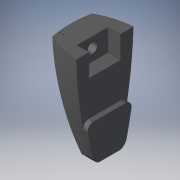
# Autodesk Inventor part: SCHUNK-1012602-FIN Co-act EGP 40/12
Saved by Autodesk Inventor 2019 (Build 230136000, 136)
## iProperties
Created: 2022-08-31
Part Number: SCHUNK-1012602-FIN Co-act EGP 40/12
Material: Generic
Catalog Web Link: www.cadenas.de
Description: FIN Co-act EGP-Finger Co-act EGP
Vendor: SCHUNK
Document SubType Name: Modeling
Designer: psAdmin
Manufacturer: SCHUNK
Mass: 14.2993 g
Surface Area: 56.9763 cm^2
Volume: 14.2993 cm^3
Density: 1 g/cm^3
Appearance: PSOLRGB-229-229-229
Category: PARTsolutions
Company: SCHUNK
Title: SCHUNK-1012602-FIN Co-act EGP 40/12
Author: Cadenas PARTsolutions
Comments: Finger Co-act EGP
PSOL_IDENT_0: {$CADENAS_DATA/23d-libs/schunk/greifsysteme/greifmodule/co_act/co_act_egp_c/fin_co_act_egp.prj},218
PSOL_IDENT_1: {VTYP=3D},{NB=SCHUNK-1012602-FIN Co-act EGP 40/12},{LINA=SCHUNK-1012602-FIN Co-act EGP 40/12},{NN=FI
PSOL_IDENT_2: N Co-act EGP},{DATE=21.12.2021 12:22:33},{GEOMDATE=21.11.2019 10:27:04},{VERSION=},{LINEID=30},{WBVA
PSOL_IDENT_3: R=},{WBNUMERIC=}  {NB=SCHUNK-1012602-FIN Co-act EGP 40/12},{LINA=SCHUNK-1012602-FIN Co-act EGP 40/12
PSOL_IDENT_4: },{KT=DUMMY},{IDNR=1012602},{TYP=FIN Co-act EGP 40/12},{TYP1=1.000},{R1=96.286},{L1=14.000},{A1=20.5
PSOL_IDENT_5: 00},{A2=0.000},{A3=0.000},{PARTSERVER=1},{B=0.000},{ANFGPKTEGH=0.000}
NB: SCHUNK-1012602-FIN Co-act EGP 40/12
NN: FIN Co-act EGP
NT: Finger Co-act EGP
NBSYN: SCHUNK-$IDNR.-$TYP.
LINA: SCHUNK-1012602-FIN Co-act EGP 40/12
CATALOG: SCHUNK
IDNR: 1012602
TYP: FIN Co-act EGP 40/12
TYP1: 1
R1: 96.286
L1: 14
A1: 20.5
A2: 0
A3: 0
PARTSERVER: 1
B: 0
ANFGPKTEGH: 0
SUPPLIER: SCHUNK
ARTICLENO: SCHUNK-1012602-FIN Co-act EGP 40/12
BOMINFO: SCHUNK-1012602-FIN Co-act EGP 40/12
CREATOR: CADENAS GmbH
Autodesk Inventor part; units mm, degrees
sketch "Sketch_1" plane through (0, 0, 0) normal (0, 0, 1) x (1, 0, 0)
  line L0 (0, 50) -> (0, 0)
  line L1 (0, 0) -> (20.15, 0)
  arc A0 (20.15, 0) -> (20.5, 0.35) centre (20.15, 0.35) ccw
  line L2 (20.5, 0.35) -> (20.5, 50)
  line L3 (20.5, 50) -> (0, 50)
  constraints: 8 end point, 2 point on circle, 1 centre point
extrude "Extrusion1" add sketch "Sketch_1" along normal mid plane 30
sketch "Sketch_2" plane through (0, 0, 0) normal (0, 0, 1) x (1, 0, 0)
  line L0 (18, 50) -> (18, 20.0436)
  line L1 (18, 20.0436) -> (20.5, 20)
  line L2 (20.5, 20) -> (20.5, 50)
  line L3 (20.5, 50) -> (18, 50)
  constraints: 8 end point
extrude "Extrusion2" cut sketch "Sketch_2" along normal mid plane 30
sketch "Sketch_4" plane through (0, 0, 0) normal (0, 0, 1) x (1, 0, 0)
  line L0 (49.5, 60) -> (49.5, -60)
  line L1 (-6, 50) -> (-6, 0)
  line L2 (-6, 0) -> (14, 0)
  arc A0 (0, 50) -> (14, 0) centre (96.286, 50.0001) ccw
  line L3 (0, 50) -> (-6, 50)
  constraints: 8 end point, 2 point on circle, 1 centre point
revolve "Revolution1" cut sketch "Sketch_4" angle 55 mid plane about axis through (49.5, 60, 0) along (0, -1, 0)
sketch "Sketch_5" plane through (20.5, 0, 0) normal (1, 0, 0) x (0, 0, -1)
  line L0 (28, 60) -> (28, -60)
  line L1 (-28, 50) -> (-28, 0)
  line L2 (-28, 0) -> (-8, 0)
  arc A0 (-12, 20) -> (-8, 0) centre (284.0042, 68.8008) ccw
  arc A1 (-15, 50) -> (-12, 20) centre (221.5611, 58.5061) ccw
  line L3 (-15, 50) -> (-28, 50)
  constraints: 8 end point, 4 point on circle, 2 centre point
revolve "Revolution2" cut sketch "Sketch_5" angle 360 about axis through (20.5, 60, -28) along (0, 1, 0)
sketch "Sketch_6" plane through (20.5, 0, 0) normal (1, 0, 0) x (0, 0, -1)
  line L0 (-28, -60) -> (-28, 60)
  line L1 (8, 0) -> (28, 0)
  line L2 (28, 0) -> (28, 50)
  line L3 (28, 50) -> (15, 50)
  arc A0 (12, 20) -> (15, 50) centre (-221.5611, 58.5061) ccw
  arc A1 (8, 0) -> (12, 20) centre (-284.0042, 68.8008) ccw
  constraints: 8 end point, 4 point on circle, 2 centre point
revolve "Revolution3" cut sketch "Sketch_6" angle 360 about axis through (20.5, -60, 28) along (0, -1, 0)
sketch "Sketch_7" plane through (0, 0, 0) normal (0, 0, 1) x (1, 0, 0)
  line L0 (11.5, 38.4) -> (20.5, 38.4)
  line L1 (20.5, 38.4) -> (20.5, 50)
  line L2 (20.5, 50) -> (11.5, 50)
  line L3 (11.5, 50) -> (11.5, 38.4)
  constraints: 8 end point
extrude "Extrusion3" cut sketch "Sketch_7" along normal mid plane 16.2
sketch "Sketch_3" plane through (0, 0, 0) normal (1, 0, 0) x (0, 1, 0)
  line L0 (50, 6.6105) -> (5.9632, 3.7355)
  arc A0 (5.9632, 3.7355) -> (5.9632, -3.7355) centre (10, 0) ccw
  line L1 (5.9632, -3.7355) -> (50, -6.6105)
  line L2 (50, -6.6105) -> (50, -6.4925)
  line L3 (50, -6.4925) -> (6.0208, -3.6505)
  arc A1 (6.0208, 3.6505) -> (6.0208, -3.6505) centre (10, 0) ccw
  line L4 (6.0208, 3.6505) -> (50, 6.4925)
  line L5 (50, 6.4925) -> (50, 6.6105)
  constraints: 12 end point, 4 point on circle, 2 centre point
extrude "Extrusion4" cut sketch "Sketch_3" along normal blind 12
sketch "Sketch_10" plane through (11.5, 0, 0) normal (1, 0, 0) x (0, 0, -1)
  line L0 (-6.6105, 50) -> (-5.8532, 38.4)
  line L1 (-5.8532, 38.4) -> (5.8532, 38.4)
  line L2 (5.8532, 38.4) -> (6.6105, 50)
  line L3 (6.6105, 50) -> (6.4925, 50)
  line L4 (6.4925, 50) -> (5.7494, 38.5)
  line L5 (5.7494, 38.5) -> (-5.7494, 38.5)
  line L6 (-5.7494, 38.5) -> (-6.4925, 50)
  line L7 (-6.4925, 50) -> (-6.6105, 50)
  constraints: 16 end point
extrude "Extrusion5" add sketch "Sketch_10" against normal blind 8
sketch "Sketch_8" plane through (0, 0, 0) normal (0, 0, 1) x (1, 0, 0)
  line L0 (11.5, 44.5) -> (0, 44.5)
  line L1 (0, 44.5) -> (0, 47)
  line L2 (0, 47) -> (2, 47)
  line L3 (2, 47) -> (2, 49)
  line L4 (2, 49) -> (7.75, 49)
  line L5 (7.75, 49) -> (7.75, 47.1)
  line L6 (7.75, 47.1) -> (11.5, 47.1)
  line L7 (11.5, 47.1) -> (11.5, 44.5)
  line L8 (11.5, 44.5) -> (0, 44.5)
  constraints: 18 end point
revolve "Revolution4" cut sketch "Sketch_8" angle 360 about axis through (11.5, 44.5, 0) along (1, 0, 0)
sketch "Sketch_13" plane through (0, 0, 0) normal (0, 0, 1) x (1, 0, 0)
  line L0 (0, 0.3578) -> (0, 0)
  line L1 (0, 0) -> (20.5, 0)
  line L2 (20.5, 0) -> (0, 0.3578)
  constraints: 6 end point
extrude "Extrusion6" cut sketch "Sketch_13" along normal mid plane 30
sketch "Sketch_15" plane through (0, 0, 0) normal (0, 0, 1) x (1, 0, 0)
  line L0 (53.5, 60) -> (53.5, -60)
  line L1 (-6, 50) -> (-6, 0)
  line L2 (-6, 0) -> (17.4472, 0)
  arc A0 (12.2079, 3.076) -> (17.4472, 0) centre (17.4472, 6) ccw
  arc A1 (0, 50) -> (12.2079, 3.076) centre (96.286, 50.0001) ccw
  line L3 (0, 50) -> (-6, 50)
  constraints: 8 end point, 4 point on circle, 2 centre point
revolve "Revolution5" cut sketch "Sketch_15" angle 360 about axis through (53.5, 60, 0) along (0, 1, 0)
fillet "Fillet1" radius 3.1 2 edges at (19.2494, 20.0218, -11.984) (19.2494, 20.0218, 11.984)
sketch "Sketch_16" plane through (20.5, 0, 0) normal (1, 0, 0) x (0, 0, -1)
  line L0 (8.1, 38.4) -> (8.3025, 38.4)
  line L1 (8.3025, 38.4) -> (8.1, 50)
  line L2 (8.1, 50) -> (8.1, 38.4)
  constraints: 6 end point
extrude "Extrusion7" cut sketch "Sketch_16" against normal blind 9
sketch "Sketch_17" plane through (20.5, 0, 0) normal (1, 0, 0) x (0, 0, -1)
  line L0 (-8.3025, 38.4) -> (-8.1, 38.4)
  line L1 (-8.1, 38.4) -> (-8.1, 50)
  line L2 (-8.1, 50) -> (-8.3025, 38.4)
  constraints: 6 end point
extrude "Extrusion8" cut sketch "Sketch_17" against normal blind 9
sketch "Sketch_18" plane through (0, 0, 0) normal (0, 0, 1) x (1, 0, 0)
  line L0 (11.5, 38.4) -> (18, 38.2865)
  line L1 (18, 38.2865) -> (18, 38.4)
  line L2 (18, 38.4) -> (11.5, 38.4)
  constraints: 6 end point
extrude "Extrusion9" cut sketch "Sketch_18" along normal mid plane 16.605
sketch "Sketch_19" plane through (0, 0, 0) normal (0, 0, 1) x (1, 0, 0)
  line L0 (0, 49.6858) -> (18, 50)
  line L1 (18, 50) -> (0, 50)
  line L2 (0, 50) -> (0, 49.6858)
  constraints: 6 end point
extrude "Extrusion10" cut sketch "Sketch_19" along normal mid plane 30
sketch "Sketch_9" plane through (20.5, 0, 0) normal (1, 0, 0) x (0, 0, -1)
  arc A0 (-8.8956, 3.9186) -> (-8, 0) centre (284.0042, 68.8008) ccw
  line L0 (-8, 0) -> (-4.014, 0)
  arc A1 (-8.8956, 3.9186) -> (-4.014, 0) centre (-4.014, 5) ccw
  constraints: 4 point on circle, 2 centre point, 2 end point
extrude "Extrusion11" cut sketch "Sketch_9" against normal blind 15
sketch "Sketch_11" plane through (20.5, 0, 0) normal (1, 0, 0) x (0, 0, -1)
  line L0 (4.014, 0) -> (8, 0)
  arc A0 (8, 0) -> (8.8956, 3.9186) centre (-284.0042, 68.8008) ccw
  arc A1 (4.014, 0) -> (8.8956, 3.9186) centre (4.014, 5) ccw
  constraints: 4 point on circle, 2 centre point, 2 end point
extrude "Extrusion12" cut sketch "Sketch_11" against normal blind 15
ref_plane "AUB_XY" through (20.5, 10, 0) normal (1, 0, 0) x (0, 0, -1)
ref_plane "AUB_YZ" through (20.5, 10, 0) normal (0, 0, -1) x (0, 1, 0)
ref_plane "AUB_ZX" through (20.5, 10, 0) normal (0, 1, 0) x (1, 0, 0)
ref_plane "AUB_DUMMY_XY" through (0, 0, 0) normal (0, 1, 0) x (1, 0, 0)
ref_plane "AUB_DUMMY_YZ" through (0, 0, 0) normal (1, 0, 0) x (0, 0, -1)
ref_plane "AUB_DUMMY_ZX" through (0, 0, 0) normal (0, 0, -1) x (0, 1, 0)
ref_plane "FIN_XY" through (11.5, 38.4, 0) normal (1, 0, 0) x (0, 0, -1)
ref_plane "FIN_YZ" through (11.5, 38.4, 0) normal (0, 0, -1) x (0, 1, 0)
ref_plane "FIN_ZX" through (11.5, 38.4, 0) normal (0, 1, 0) x (1, 0, 0)
body "Solid1"
